Autodesk Fusion 360 part; units mm, degrees
(part 2 of 2)
  spline S17 degree 5 poles (-58.6418, 16.0133) (-58.6497, 16.0148) (-58.6655, 16.0179) (-58.6891, 16.0234) (-58.7202, 16.0321) (-58.7585, 16.0449) (-58.7966, 16.0592) (-58.8344, 16.0742) (-58.8721, 16.0898) (-58.9098, 16.1057) (-58.9473, 16.1219) (-58.9848, 16.1386) (-59.0221, 16.1559) (-59.0592, 16.1739) (-59.0961, 16.1925) (-59.1328, 16.2118) (-59.1694, 16.2316) (-59.2058, 16.2519) (-59.2421, 16.2725) (-59.2783, 16.2936) (-59.3144, 16.315) (-59.3503, 16.3368) (-59.3861, 16.3591) (-59.4217, 16.3818) (-59.4572, 16.4049) (-59.4926, 16.4284) (-59.5278, 16.4523) (-59.5629, 16.4765) (-59.5978, 16.5011) (-59.6326, 16.5261) (-59.6673, 16.5514) (-59.7019, 16.577) (-59.7363, 16.603) (-59.7705, 16.6293) (-59.8047, 16.656) (-59.8387, 16.683) (-59.8725, 16.7103) (-59.9063, 16.738) (-59.9399, 16.766) (-59.9733, 16.7942) (-60.0066, 16.8228) (-60.0398, 16.8517) (-60.0728, 16.8809) (-60.1057, 16.9103) (-60.1385, 16.9401) (-60.1711, 16.9702) (-60.2036, 17.0006) (-60.2359, 17.0312) (-60.2681, 17.0621) (-60.3001, 17.0933) (-60.332, 17.1248) (-60.3638, 17.1566) (-60.3954, 17.1886) (-60.4269, 17.2209) (-60.4582, 17.2535) (-60.4894, 17.2863) (-60.5204, 17.3194) (-60.5513, 17.3528) (-60.5821, 17.3864) (-60.6126, 17.4203) (-60.6431, 17.4544) (-60.6734, 17.4888) (-60.7035, 17.5235) (-60.7335, 17.5584) (-60.7634, 17.5935) (-60.7931, 17.6289) (-60.8226, 17.6645) (-60.852, 17.7004) (-60.8812, 17.7365) (-60.9103, 17.7728) (-60.9392, 17.8094) (-60.9622, 17.8388) (-60.9794, 17.861) (-60.9909, 17.8759) (-60.9966, 17.8833) knots 0 0 0 0 0 0 0.01428571 0.02857143 0.04285714 0.05714286 0.07142857 0.08571429 0.1 0.11428571 0.12857143 0.14285714 0.15714286 0.17142857 0.18571429 0.2 0.21428571 0.22857143 0.24285714 0.25714286 0.27142857 0.28571429 0.3 0.31428571 0.32857143 0.34285714 0.35714286 0.37142857 0.38571429 0.4 0.41428571 0.42857143 0.44285714 0.45714286 0.47142857 0.48571429 0.5 0.51428571 0.52857143 0.54285714 0.55714286 0.57142857 0.58571429 0.6 0.61428571 0.62857143 0.64285714 0.65714286 0.67142857 0.68571429 0.7 0.71428571 0.72857143 0.74285714 0.75714286 0.77142857 0.78571429 0.8 0.81428571 0.82857143 0.84285714 0.85714286 0.87142857 0.88571429 0.9 0.91428571 0.92857143 0.94285714 0.95714286 0.97142857 0.98571429 1 1 1 1 1 1
  line L17 (-58.6418, 16.0133) -> (-57.3735, 15.7814)
  arc A35 (-56.9677, 15.2247) -> (-57.3735, 15.7814) centre (-57.4635, 15.2895) ccw
  arc A36 (-56.9677, 15.2247) -> (-57.0478, 13.9766) centre (-47.5478, 13.9934) ccw
  arc A37 (-57.5215, 13.4765) -> (-57.0478, 13.9766) centre (-57.5478, 13.9758) ccw
  line L18 (-57.5215, 13.4765) -> (-58.809, 13.4086)
  spline S18 degree 5 poles (-58.809, 13.4086) (-58.817, 13.4081) (-58.8331, 13.407) (-58.8572, 13.4046) (-58.8891, 13.3999) (-58.9288, 13.3921) (-58.9684, 13.3829) (-59.0078, 13.3728) (-59.0472, 13.3622) (-59.0866, 13.3512) (-59.1259, 13.3399) (-59.1652, 13.3282) (-59.2044, 13.3158) (-59.2435, 13.3027) (-59.2825, 13.2889) (-59.3214, 13.2745) (-59.3602, 13.2595) (-59.3989, 13.2441) (-59.4375, 13.2282) (-59.4761, 13.212) (-59.5146, 13.1953) (-59.553, 13.1783) (-59.5914, 13.1608) (-59.6296, 13.1429) (-59.6678, 13.1245) (-59.7059, 13.1057) (-59.7438, 13.0865) (-59.7817, 13.0669) (-59.8195, 13.047) (-59.8573, 13.0267) (-59.8949, 13.006) (-59.9324, 12.985) (-59.9699, 12.9637) (-60.0073, 12.9419) (-60.0445, 12.9198) (-60.0817, 12.8974) (-60.1188, 12.8746) (-60.1557, 12.8515) (-60.1926, 12.8281) (-60.2294, 12.8043) (-60.2661, 12.7802) (-60.3027, 12.7558) (-60.3392, 12.7311) (-60.3756, 12.7061) (-60.4119, 12.6807) (-60.4481, 12.6551) (-60.4842, 12.6291) (-60.5202, 12.6029) (-60.556, 12.5763) (-60.5918, 12.5494) (-60.6275, 12.5223) (-60.663, 12.4949) (-60.6985, 12.4671) (-60.7338, 12.4391) (-60.7691, 12.4108) (-60.8042, 12.3822) (-60.8392, 12.3534) (-60.8741, 12.3242) (-60.9089, 12.2948) (-60.9436, 12.2651) (-60.9781, 12.2352) (-61.0126, 12.2049) (-61.0469, 12.1744) (-61.0811, 12.1436) (-61.1152, 12.1126) (-61.1492, 12.0813) (-61.183, 12.0498) (-61.2168, 12.018) (-61.2504, 11.9859) (-61.2838, 11.9536) (-61.3172, 11.921) (-61.3438, 11.8947) (-61.3637, 11.8749) (-61.3769, 11.8616) (-61.3835, 11.855) knots 0 0 0 0 0 0 0.01428571 0.02857143 0.04285714 0.05714286 0.07142857 0.08571429 0.1 0.11428571 0.12857143 0.14285714 0.15714286 0.17142857 0.18571429 0.2 0.21428571 0.22857143 0.24285714 0.25714286 0.27142857 0.28571429 0.3 0.31428571 0.32857143 0.34285714 0.35714286 0.37142857 0.38571429 0.4 0.41428571 0.42857143 0.44285714 0.45714286 0.47142857 0.48571429 0.5 0.51428571 0.52857143 0.54285714 0.55714286 0.57142857 0.58571429 0.6 0.61428571 0.62857143 0.64285714 0.65714286 0.67142857 0.68571429 0.7 0.71428571 0.72857143 0.74285714 0.75714286 0.77142857 0.78571429 0.8 0.81428571 0.82857143 0.84285714 0.85714286 0.87142857 0.88571429 0.9 0.91428571 0.92857143 0.94285714 0.95714286 0.97142857 0.98571429 1 1 1 1 1 1
  arc A38 (-61.3835, 11.855) -> (-61.1397, 10.6378) centre (-47.5478, 13.9934) ccw
  spline S19 degree 5 poles (-58.1654, 10.1957) (-58.173, 10.193) (-58.1883, 10.1878) (-58.2115, 10.1808) (-58.2427, 10.1728) (-58.2823, 10.1647) (-58.3224, 10.158) (-58.3627, 10.1522) (-58.4031, 10.1468) (-58.4437, 10.1417) (-58.4843, 10.137) (-58.5251, 10.1327) (-58.5661, 10.129) (-58.6072, 10.1261) (-58.6485, 10.1237) (-58.6899, 10.1221) (-58.7315, 10.121) (-58.7732, 10.1203) (-58.8149, 10.1201) (-58.8568, 10.1202) (-58.8987, 10.1207) (-58.9408, 10.1217) (-58.9829, 10.123) (-59.0251, 10.1248) (-59.0674, 10.1271) (-59.1097, 10.1298) (-59.1522, 10.1329) (-59.1947, 10.1363) (-59.2373, 10.1402) (-59.2799, 10.1444) (-59.3226, 10.1489) (-59.3653, 10.1539) (-59.4081, 10.1592) (-59.451, 10.1648) (-59.4939, 10.1709) (-59.5368, 10.1773) (-59.5798, 10.184) (-59.6228, 10.1911) (-59.6659, 10.1985) (-59.709, 10.2062) (-59.7521, 10.2143) (-59.7953, 10.2228) (-59.8385, 10.2315) (-59.8817, 10.2406) (-59.925, 10.25) (-59.9683, 10.2597) (-60.0116, 10.2698) (-60.0549, 10.2802) (-60.0982, 10.2909) (-60.1416, 10.3019) (-60.185, 10.3132) (-60.2284, 10.3248) (-60.2718, 10.3368) (-60.3152, 10.349) (-60.3586, 10.3615) (-60.402, 10.3744) (-60.4454, 10.3875) (-60.4889, 10.401) (-60.5323, 10.4147) (-60.5757, 10.4288) (-60.6192, 10.4431) (-60.6626, 10.4578) (-60.706, 10.4727) (-60.7494, 10.4879) (-60.7929, 10.5034) (-60.8363, 10.5192) (-60.8797, 10.5353) (-60.923, 10.5517) (-60.9664, 10.5683) (-61.0098, 10.5852) (-61.0531, 10.6025) (-61.0878, 10.6164) (-61.1137, 10.6271) (-61.1311, 10.6342) (-61.1397, 10.6378) knots 0 0 0 0 0 0 0.01428571 0.02857143 0.04285714 0.05714286 0.07142857 0.08571429 0.1 0.11428571 0.12857143 0.14285714 0.15714286 0.17142857 0.18571429 0.2 0.21428571 0.22857143 0.24285714 0.25714286 0.27142857 0.28571429 0.3 0.31428571 0.32857143 0.34285714 0.35714286 0.37142857 0.38571429 0.4 0.41428571 0.42857143 0.44285714 0.45714286 0.47142857 0.48571429 0.5 0.51428571 0.52857143 0.54285714 0.55714286 0.57142857 0.58571429 0.6 0.61428571 0.62857143 0.64285714 0.65714286 0.67142857 0.68571429 0.7 0.71428571 0.72857143 0.74285714 0.75714286 0.77142857 0.78571429 0.8 0.81428571 0.82857143 0.84285714 0.85714286 0.87142857 0.88571429 0.9 0.91428571 0.92857143 0.94285714 0.95714286 0.97142857 0.98571429 1 1 1 1 1 1
  line L19 (-58.1654, 10.1957) -> (-56.9511, 10.629)
  arc A39 (-56.3213, 10.3498) -> (-56.9511, 10.629) centre (-56.7831, 10.1581) ccw
  arc A40 (-56.3213, 10.3498) -> (-55.7667, 9.2289) centre (-47.5478, 13.9934) ccw
  arc A41 (-55.9268, 8.5589) -> (-55.7667, 9.2289) centre (-56.1992, 8.9781) ccw
  line L20 (-55.9268, 8.5589) -> (-57.0078, 7.8563)
  spline S20 degree 5 poles (-57.0078, 7.8563) (-57.0146, 7.8519) (-57.028, 7.8429) (-57.0476, 7.8288) (-57.073, 7.8088) (-57.1034, 7.7822) (-57.133, 7.7544) (-57.1621, 7.7259) (-57.191, 7.6971) (-57.2196, 7.6679) (-57.248, 7.6384) (-57.2761, 7.6086) (-57.3039, 7.5783) (-57.3312, 7.5474) (-57.3581, 7.516) (-57.3846, 7.4841) (-57.4107, 7.4517) (-57.4365, 7.4189) (-57.462, 7.3859) (-57.4873, 7.3525) (-57.5123, 7.3189) (-57.5371, 7.2849) (-57.5615, 7.2506) (-57.5857, 7.2159) (-57.6096, 7.1809) (-57.6331, 7.1456) (-57.6564, 7.11) (-57.6795, 7.0741) (-57.7022, 7.0379) (-57.7247, 7.0015) (-57.747, 6.9648) (-57.769, 6.9278) (-57.7908, 6.8906) (-57.8123, 6.8531) (-57.8335, 6.8153) (-57.8545, 6.7773) (-57.8752, 6.739) (-57.8957, 6.7005) (-57.9159, 6.6618) (-57.9359, 6.6228) (-57.9556, 6.5836) (-57.9751, 6.5442) (-57.9943, 6.5045) (-58.0133, 6.4647) (-58.0321, 6.4246) (-58.0506, 6.3843) (-58.0689, 6.3437) (-58.0869, 6.303) (-58.1047, 6.2621) (-58.1223, 6.2209) (-58.1396, 6.1796) (-58.1567, 6.138) (-58.1735, 6.0963) (-58.1901, 6.0543) (-58.2065, 6.0122) (-58.2226, 5.9699) (-58.2385, 5.9274) (-58.2541, 5.8847) (-58.2695, 5.8418) (-58.2847, 5.7988) (-58.2997, 5.7556) (-58.3144, 5.7122) (-58.3289, 5.6686) (-58.3431, 5.6248) (-58.3571, 5.5809) (-58.3709, 5.5368) (-58.3844, 5.4926) (-58.3977, 5.4482) (-58.4108, 5.4036) (-58.4236, 5.3588) (-58.4362, 5.3139) (-58.4461, 5.2779) (-58.4535, 5.2508) (-58.4583, 5.2327) (-58.4607, 5.2236) knots 0 0 0 0 0 0 0.01428571 0.02857143 0.04285714 0.05714286 0.07142857 0.08571429 0.1 0.11428571 0.12857143 0.14285714 0.15714286 0.17142857 0.18571429 0.2 0.21428571 0.22857143 0.24285714 0.25714286 0.27142857 0.28571429 0.3 0.31428571 0.32857143 0.34285714 0.35714286 0.37142857 0.38571429 0.4 0.41428571 0.42857143 0.44285714 0.45714286 0.47142857 0.48571429 0.5 0.51428571 0.52857143 0.54285714 0.55714286 0.57142857 0.58571429 0.6 0.61428571 0.62857143 0.64285714 0.65714286 0.67142857 0.68571429 0.7 0.71428571 0.72857143 0.74285714 0.75714286 0.77142857 0.78571429 0.8 0.81428571 0.82857143 0.84285714 0.85714286 0.87142857 0.88571429 0.9 0.91428571 0.92857143 0.94285714 0.95714286 0.97142857 0.98571429 1 1 1 1 1 1
  arc A42 (-58.4607, 5.2236) -> (-57.6409, 4.2914) centre (-47.5478, 13.9934) ccw
  spline S21 degree 5 poles (-54.8441, 5.3958) (-54.8493, 5.3896) (-54.86, 5.3775) (-54.8765, 5.3598) (-54.8996, 5.3372) (-54.9298, 5.3104) (-54.9612, 5.2846) (-54.9931, 5.2594) (-55.0255, 5.2345) (-55.0581, 5.2098) (-55.0909, 5.1854) (-55.1241, 5.1613) (-55.1577, 5.1377) (-55.1918, 5.1145) (-55.2264, 5.0919) (-55.2615, 5.0697) (-55.2969, 5.0479) (-55.3327, 5.0265) (-55.3687, 5.0054) (-55.4051, 4.9846) (-55.4416, 4.9641) (-55.4785, 4.9439) (-55.5157, 4.924) (-55.5531, 4.9045) (-55.5909, 4.8853) (-55.6289, 4.8665) (-55.6672, 4.8479) (-55.7058, 4.8296) (-55.7445, 4.8117) (-55.7836, 4.794) (-55.8228, 4.7766) (-55.8623, 4.7595) (-55.902, 4.7427) (-55.942, 4.7262) (-55.9821, 4.71) (-56.0225, 4.694) (-56.0631, 4.6784) (-56.1039, 4.663) (-56.1449, 4.6479) (-56.1861, 4.633) (-56.2275, 4.6185) (-56.2691, 4.6042) (-56.3109, 4.5902) (-56.3529, 4.5764) (-56.3951, 4.563) (-56.4374, 4.5497) (-56.4799, 4.5368) (-56.5226, 4.5241) (-56.5655, 4.5117) (-56.6086, 4.4996) (-56.6518, 4.4877) (-56.6952, 4.4761) (-56.7387, 4.4647) (-56.7825, 4.4536) (-56.8263, 4.4427) (-56.8704, 4.4322) (-56.9145, 4.4218) (-56.9589, 4.4118) (-57.0034, 4.402) (-57.048, 4.3924) (-57.0928, 4.3831) (-57.1377, 4.3741) (-57.1828, 4.3653) (-57.228, 4.3567) (-57.2734, 4.3485) (-57.3188, 4.3404) (-57.3645, 4.3327) (-57.4102, 4.3252) (-57.4561, 4.3179) (-57.5021, 4.3109) (-57.5482, 4.3041) (-57.5853, 4.2989) (-57.6131, 4.2951) (-57.6316, 4.2926) (-57.6409, 4.2914) knots 0 0 0 0 0 0 0.01428571 0.02857143 0.04285714 0.05714286 0.07142857 0.08571429 0.1 0.11428571 0.12857143 0.14285714 0.15714286 0.17142857 0.18571429 0.2 0.21428571 0.22857143 0.24285714 0.25714286 0.27142857 0.28571429 0.3 0.31428571 0.32857143 0.34285714 0.35714286 0.37142857 0.38571429 0.4 0.41428571 0.42857143 0.44285714 0.45714286 0.47142857 0.48571429 0.5 0.51428571 0.52857143 0.54285714 0.55714286 0.57142857 0.58571429 0.6 0.61428571 0.62857143 0.64285714 0.65714286 0.67142857 0.68571429 0.7 0.71428571 0.72857143 0.74285714 0.75714286 0.77142857 0.78571429 0.8 0.81428571 0.82857143 0.84285714 0.85714286 0.87142857 0.88571429 0.9 0.91428571 0.92857143 0.94285714 0.95714286 0.97142857 0.98571429 1 1 1 1 1 1
  line L21 (-54.8441, 5.3958) -> (-54.0091, 6.3781)
  arc A43 (-53.3241, 6.4512) -> (-54.0091, 6.3781) centre (-53.6281, 6.0543) ccw
  arc A44 (-53.3241, 6.4512) -> (-52.2833, 5.7578) centre (-47.5478, 13.9934) ccw
  arc A45 (-52.0869, 5.0975) -> (-52.2833, 5.7578) centre (-52.5325, 5.3244) ccw
  line L22 (-52.0869, 5.0975) -> (-52.6719, 3.9486)
  spline S22 degree 5 poles (-52.6719, 3.9486) (-52.6755, 3.9414) (-52.6826, 3.9269) (-52.6926, 3.9048) (-52.7045, 3.8748) (-52.7176, 3.8365) (-52.7294, 3.7977) (-52.7403, 3.7585) (-52.7508, 3.719) (-52.761, 3.6795) (-52.7709, 3.6398) (-52.7804, 3.5999) (-52.7893, 3.5597) (-52.7975, 3.5193) (-52.8051, 3.4787) (-52.812, 3.4378) (-52.8184, 3.3967) (-52.8244, 3.3554) (-52.83, 3.314) (-52.8352, 3.2725) (-52.8401, 3.2308) (-52.8445, 3.189) (-52.8485, 3.1471) (-52.8521, 3.105) (-52.8553, 3.0628) (-52.8581, 3.0204) (-52.8604, 2.9779) (-52.8624, 2.9353) (-52.8641, 2.8926) (-52.8653, 2.8498) (-52.8663, 2.8069) (-52.8668, 2.7638) (-52.867, 2.7207) (-52.8669, 2.6775) (-52.8664, 2.6342) (-52.8656, 2.5908) (-52.8644, 2.5473) (-52.8629, 2.5037) (-52.861, 2.46) (-52.8588, 2.4163) (-52.8563, 2.3725) (-52.8535, 2.3286) (-52.8503, 2.2846) (-52.8468, 2.2406) (-52.843, 2.1965) (-52.8389, 2.1523) (-52.8345, 2.1081) (-52.8297, 2.0638) (-52.8247, 2.0194) (-52.8193, 1.975) (-52.8136, 1.9305) (-52.8076, 1.886) (-52.8013, 1.8415) (-52.7948, 1.7968) (-52.7879, 1.7522) (-52.7807, 1.7075) (-52.7732, 1.6627) (-52.7654, 1.6179) (-52.7573, 1.5731) (-52.7489, 1.5282) (-52.7403, 1.4833) (-52.7313, 1.4384) (-52.7221, 1.3934) (-52.7125, 1.3484) (-52.7027, 1.3033) (-52.6926, 1.2583) (-52.6822, 1.2132) (-52.6715, 1.1681) (-52.6605, 1.1229) (-52.6493, 1.0777) (-52.6377, 1.0326) (-52.6283, 0.9964) (-52.6211, 0.9693) (-52.6162, 0.9512) (-52.6138, 0.9421) knots 0 0 0 0 0 0 0.01428571 0.02857143 0.04285714 0.05714286 0.07142857 0.08571429 0.1 0.11428571 0.12857143 0.14285714 0.15714286 0.17142857 0.18571429 0.2 0.21428571 0.22857143 0.24285714 0.25714286 0.27142857 0.28571429 0.3 0.31428571 0.32857143 0.34285714 0.35714286 0.37142857 0.38571429 0.4 0.41428571 0.42857143 0.44285714 0.45714286 0.47142857 0.48571429 0.5 0.51428571 0.52857143 0.54285714 0.55714286 0.57142857 0.58571429 0.6 0.61428571 0.62857143 0.64285714 0.65714286 0.67142857 0.68571429 0.7 0.71428571 0.72857143 0.74285714 0.75714286 0.77142857 0.78571429 0.8 0.81428571 0.82857143 0.84285714 0.85714286 0.87142857 0.88571429 0.9 0.91428571 0.92857143 0.94285714 0.95714286 0.97142857 0.98571429 1 1 1 1 1 1
  arc A46 (-52.6138, 0.9421) -> (-51.4377, 0.5447) centre (-47.5478, 13.9934) ccw
  spline S23 degree 5 poles (-49.5677, 2.8995) (-49.5692, 2.8915) (-49.5723, 2.8757) (-49.5778, 2.8521) (-49.5865, 2.8211) (-49.5993, 2.7827) (-49.6136, 2.7447) (-49.6286, 2.7069) (-49.6442, 2.6691) (-49.6601, 2.6315) (-49.6763, 2.5939) (-49.693, 2.5565) (-49.7103, 2.5192) (-49.7283, 2.4821) (-49.7469, 2.4452) (-49.7662, 2.4084) (-49.786, 2.3719) (-49.8063, 2.3354) (-49.8269, 2.2991) (-49.848, 2.263) (-49.8694, 2.2269) (-49.8912, 2.191) (-49.9135, 2.1552) (-49.9362, 2.1195) (-49.9593, 2.084) (-49.9828, 2.0487) (-50.0067, 2.0135) (-50.0309, 1.9784) (-50.0555, 1.9434) (-50.0805, 1.9086) (-50.1058, 1.8739) (-50.1314, 1.8394) (-50.1574, 1.805) (-50.1837, 1.7707) (-50.2104, 1.7366) (-50.2374, 1.7026) (-50.2647, 1.6687) (-50.2924, 1.635) (-50.3204, 1.6014) (-50.3486, 1.5679) (-50.3772, 1.5346) (-50.4061, 1.5015) (-50.4353, 1.4684) (-50.4647, 1.4355) (-50.4945, 1.4028) (-50.5246, 1.3702) (-50.555, 1.3377) (-50.5856, 1.3054) (-50.6165, 1.2732) (-50.6477, 1.2411) (-50.6792, 1.2092) (-50.711, 1.1775) (-50.743, 1.1458) (-50.7753, 1.1144) (-50.8079, 1.083) (-50.8407, 1.0519) (-50.8738, 1.0208) (-50.9072, 0.9899) (-50.9408, 0.9592) (-50.9747, 0.9286) (-51.0088, 0.8982) (-51.0432, 0.8679) (-51.0779, 0.8377) (-51.1128, 0.8077) (-51.1479, 0.7779) (-51.1833, 0.7482) (-51.2189, 0.7187) (-51.2548, 0.6893) (-51.2909, 0.66) (-51.3272, 0.631) (-51.3638, 0.602) (-51.3932, 0.579) (-51.4154, 0.5618) (-51.4303, 0.5504) (-51.4377, 0.5447) knots 0 0 0 0 0 0 0.01428571 0.02857143 0.04285714 0.05714286 0.07142857 0.08571429 0.1 0.11428571 0.12857143 0.14285714 0.15714286 0.17142857 0.18571429 0.2 0.21428571 0.22857143 0.24285714 0.25714286 0.27142857 0.28571429 0.3 0.31428571 0.32857143 0.34285714 0.35714286 0.37142857 0.38571429 0.4 0.41428571 0.42857143 0.44285714 0.45714286 0.47142857 0.48571429 0.5 0.51428571 0.52857143 0.54285714 0.55714286 0.57142857 0.58571429 0.6 0.61428571 0.62857143 0.64285714 0.65714286 0.67142857 0.68571429 0.7 0.71428571 0.72857143 0.74285714 0.75714286 0.77142857 0.78571429 0.8 0.81428571 0.82857143 0.84285714 0.85714286 0.87142857 0.88571429 0.9 0.91428571 0.92857143 0.94285714 0.95714286 0.97142857 0.98571429 1 1 1 1 1 1
  line L23 (-49.5677, 2.8995) -> (-49.3358, 4.1677)
  arc A47 (-48.7791, 4.5736) -> (-49.3358, 4.1677) centre (-48.8439, 4.0778) ccw
  arc A48 (-48.7791, 4.5736) -> (-47.5311, 4.4934) centre (-47.5478, 13.9934) ccw
  circle A49 centre (-47.5478, 13.9934) radius 0.5
  circle A50 centre (-47.5478, 13.9934) radius 8
  dimension "d1" = 16
  constraint concentric A49 A50
  measures "d1" diameter of A50
move_body "Desplazar4" bodies 1 to x (1, 0, 0) y (0, 1, 0) z (0, 0, 1) at (-3, -47.5478, -13.9934)
hole "Agujero1" at (0, 0, 0) direction (-1, 0, 0) diameter 1.5 depth 11 tip angle 180 counterbore diameter 2 counterbore depth 1
hole "Agujero2" at (0, 0, 0) direction (-1, 0, 0) diameter 3 end through all
named bodies: "Engranaje motor"
